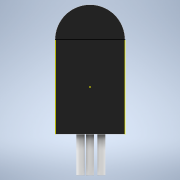
# Autodesk Inventor part: temperature sensor
Saved by Autodesk Inventor 2021 (Build 250183000, 183)
## iProperties
Created: 2021-06-29
Part Number: temperature sensor
Material: Rubber, Silicone
Document SubType Name: Modeling
Designer: HP
Density: 1.25 g/cm^3
Appearance: Rubber - Black
Author: HP
Autodesk Inventor part; units mm, degrees
ref_plane "YZ Plane" through (0, 0, 0) normal (1, 0, 0) x (0, 1, 0)
ref_plane "XZ Plane" through (0, 0, 0) normal (0, 1, 0) x (-1, 0, 0)
ref_plane "XY Plane" through (0, 0, 0) normal (0, 0, 1) x (1, 0, 0)
sketch "Sketch1" plane through (0, 0, 0) normal (0, 0, 1) x (1, 0, 0)
  line L0 (-8.5, 11.5) -> (8.5, 11.5)
  line L1 (8.5, 11.5) -> (8.5, -11.5)
  line L2 (8.5, -11.5) -> (-8.5, -11.5)
  line L3 (-8.5, -11.5) -> (-8.5, 11.5)
  line L4 (-8.5, 11.5) -> (8.5, -11.5) construction
  line L5 (8.5, 11.5) -> (-8.5, -11.5) construction
  arc A0 (8.5, 11.5) -> (-8.5, 11.5) centre (0, 11.5) ccw
  point P0 (0, 0)
  dimension "d0" = 23
  dimension "d1" = 17
  constraints: 12 end point, 2 midpoint, 2 parallel, 2 point on circle, 2 tangent, 1 centre point, 1 horizontal, 1 perpendicular
  measures "d0" distance of L0.end L1.end
  measures "d1" distance of L0.start L0.end
extrude "Extrusion1" add sketch "Sketch1" along normal blind 8
sketch "Sketch3" plane through (0, 0, 8) normal (0, 0, 1) x (1, 0, 0)
  line L0 (-8.5, 11.5) -> (-8.5, -11.5) projected
  line L1 (8.5, -11.5) -> (8.5, 11.5) projected
  line L2 (-8.5, 11.5) -> (8.5, 11.5)
  point P0 (0, 0)
  constraints: 2 end point, 1 horizontal
sketch "Sketch4" plane through (-8.5, -11.5, 0) normal (0, -1, 0) x (1, 0, 0)
  circle A0 centre (6.1706, 4.0145) radius 1
  circle A1 centre (11.2338, 3.8113) radius 1
  circle A2 centre (8.5, 3.8113) radius 1
  point P0 (8.5, 0)
  dimension "d4" = 2
  dimension "d6" = 2
  dimension "d9" = 2
  constraints: 3 centre point
  measures "d4" diameter of A0
  measures "d6" diameter of A1
  measures "d9" diameter of A2
extrude "Extrusion2" add sketch "Sketch4" along normal blind 10 contours A0 | A1
extrude "Extrusion3" add sketch "Sketch4" along normal blind 10 contours A2
body "Solid1"
